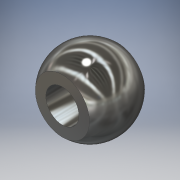
# Autodesk Inventor part: 10-32SuperDutyLinkage(Ball)-1111-2017
Saved by Autodesk Inventor 2016 SP1 (Build 200210100, 210)
## iProperties
Created: 2017-02-16
Part Number: 10-32SuperDutyLinkage(Ball)-1111-2017
Material: Stainless Steel
Document SubType Name: Modeling
Designer: 589013
Density: 8 g/cm^3
Appearance: Chrome - Polished
Author: 589013
Autodesk Inventor part; units mm, degrees
ref_plane "YZ Plane" through (0, 0, 0) normal (1, 0, 0) x (0, 1, 0)
ref_plane "XZ Plane" through (0, 0, 0) normal (0, 1, 0) x (-1, 0, 0)
ref_plane "Work Plane1" through (0, 0, -2.9766) normal (0, 0, 1) x (1, 0, 0)
sketch "Sketch1" plane through (0, 0, -2.9766) normal (0, 0, 1) x (1, 0, 0)
  line L0 (-26.9875, 5.1594) -> (-7.3502, 5.1594) construction
  spline S0 degree 3 poles (-7.3502, 5.1594) (-6.9667, 5.1594) (-6.5864, 5.2289) (-5.869, 5.5) (-5.5378, 5.6995) (-5.2502, 5.9531) knots 0 0 0 0 0.5 0.5 1 1 1 1 construction
  arc A0 (-5.2502, -5.9531) -> (-5.2502, 5.9531) centre (0, 0) ccw construction
  spline S1 degree 3 poles (-5.2502, -5.9531) (-5.5378, -5.6995) (-5.869, -5.5) (-6.5864, -5.2289) (-6.9667, -5.1594) (-7.3502, -5.1594) knots 0 0 0 0 0.5 0.5 1 1 1 1 construction
  line L1 (-7.3502, -5.1594) -> (-26.9875, -5.1594) construction
  line L2 (-26.9875, -5.1594) -> (-26.9875, -3.9688) construction
  line L3 (-26.9875, -3.9688) -> (-14.2875, -3.9688) construction
  line L4 (-14.2875, -3.9688) -> (-14.2875, 3.9687) construction
  line L5 (-14.2875, 3.9687) -> (-26.9875, 3.9687) construction
  line L6 (-26.9875, 3.9687) -> (-26.9875, 5.1594) construction
  arc A1 (0, 5.5562) -> (0, -5.5563) centre (0, 0) ccw construction
  arc A2 (0, -5.5563) -> (0, 5.5562) centre (0, 0) ccw
  line L7 (0, 5.5562) -> (0, -5.5563)
  point P0 (0, 0)
  constraints: 16 end point, 6 point on circle, 4 horizontal, 4 vertical, 3 centre point, 24 other
revolve "Revolution1" add sketch "Sketch1" angle 360 about axis through (0, 5.5562, -2.9766) along (0, -1, 0)
ref_plane "Work Plane2" through (0, 0, 0.9922) normal (0, 0, 1) x (1, 0, 0)
sketch "Sketch2" plane through (0, 0, 0.9922) normal (0, 0, 1) x (1, 0, 0)
  circle A0 centre (0, 0) radius 3.8886 projected
  point P0 (0, 0)
extrude "Extrusion1" cut sketch "Sketch2" along normal through all
mirror "Mirror1" about plane through (0, 0, -2.9766) normal (0, 0, 1) of "Extrusion1"
hole "Hole1" at (0, 0, 0.9922) direction (0, 0, -1) diameter 4.7625 end through all
body "Solid1"
